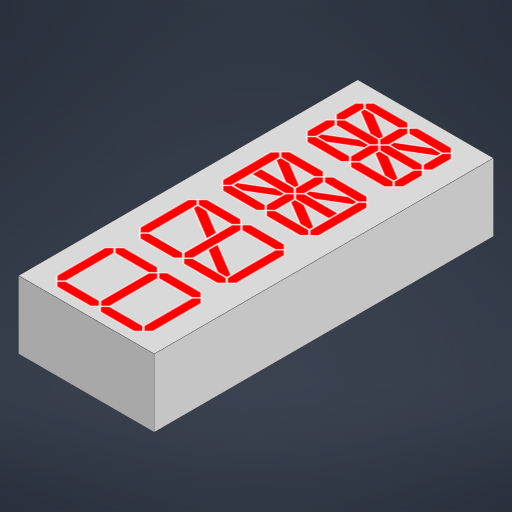
# Autodesk Inventor part: 14seg_surrogate
Saved by Autodesk Inventor 2024.2 (Build 282272000, 272)
## iProperties
Created: 2025-05-21
Part Number: 14seg_surrogate
Material: Generic
Document SubType Name: Modeling
Designer: Moe
Density: 1 g/cm^3
Appearance: Default
Author: Moe
Autodesk Inventor part; units mm, degrees
ref_plane "YZ Plane" through (0, 0, 0) normal (1, 0, 0) x (0, 1, 0)
ref_plane "XZ Plane" through (0, 0, 0) normal (0, 1, 0) x (-1, 0, 0)
ref_plane "XY Plane" through (0, 0, 0) normal (0, 0, 1) x (1, 0, 0)
sketch "Sketch1" plane through (0, 0, 0) normal (0, 1, 0) x (-1, 0, 0)
  line L0 (0, 0) -> (16, 0)
  line L1 (16, 0) -> (16, -40)
  line L2 (16, -40) -> (0, -40)
  line L3 (0, -40) -> (0, 0)
  dimension "d0" = 16
  dimension "d1" = 40
  constraints: 8 end point, 2 parallel, 1 horizontal, 1 perpendicular
  measures "d0" distance of L1.end L2.end
  measures "d1" distance of L0.end L1.end
extrude "Extrusion1" add sketch "Sketch1" along normal blind 8
sketch "Sketch2" plane through (0, 8, 0) normal (0, 1, 0) x (1, 0, 0)
  line L0 (-13.8399, 1.0329) -> (-13.8399, 38.6588) construction
  line L1 (-13.8399, 38.6588) -> (-2.21, 38.6588) construction
  line L2 (-2.21, 38.6588) -> (-2.21, 1.0329) construction
  line L3 (-2.21, 1.0329) -> (-13.8399, 1.0329) construction
  point P0 (0, 0)
  constraints: 2 other
decal "Decal1"
body "Solid1"
